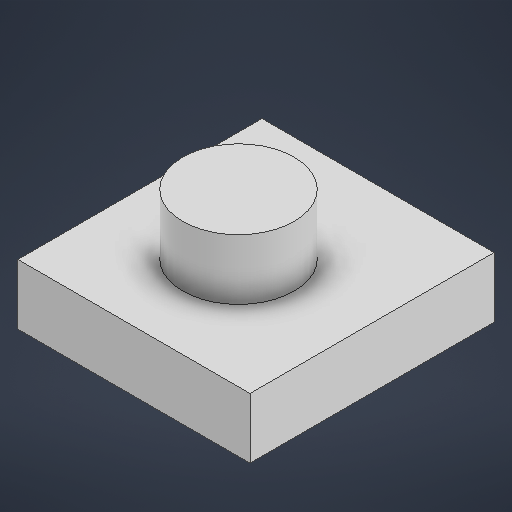
# Autodesk Inventor part: offset_sketch_plane
Saved by Autodesk Inventor 2026 (Build 300175050, 175E)
## iProperties
Created: 2025-10-13
Part Number: offset_sketch_plane
Material: Generic
Document SubType Name: Modeling
Designer: Administrator
Density: 1 g/cm^3
Appearance: Default
Author: Administrator
Autodesk Inventor part; units mm, degrees
ref_plane "YZ Plane" through (0, 0, 0) normal (1, 0, 0) x (0, 1, 0)
ref_plane "XZ Plane" through (0, 0, 0) normal (0, 1, 0) x (-1, 0, 0)
ref_plane "XY Plane" through (0, 0, 0) normal (0, 0, 1) x (1, 0, 0)
sketch "Sketch1" plane through (0, 0, 0) normal (0, 1, 0) x (-1, 0, 0)
  line L0 (0, 0) -> (9.7707, 0)
  line L1 (9.7707, 0) -> (9.7707, -10.2745)
  line L2 (9.7707, -10.2745) -> (0, -10.2745)
  line L3 (0, -10.2745) -> (0, 0)
  constraints: 8 end point, 2 parallel, 1 horizontal, 1 perpendicular
extrude "Extrusion1" add sketch "Sketch1" along normal blind 2.54
sketch "Sketch2" plane through (0, 2.54, 0) normal (0, 1, 0) x (1, 0, 0)
  circle A0 centre (-5.1463, 4.6604) radius 2.3446
  point P0 (0, 0)
  constraints: 1 centre point
extrude "Extrusion2" add sketch "Sketch2" along normal blind 2.54
body "Solid1"
